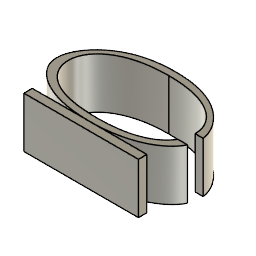
goulotte câbles (Autodesk Fusion 360 design; units mm, degrees)
Autodesk Fusion 360 part; units mm, degrees
sketch "Esquisse1" plane through (0, 0, 0) normal (0, 0, 1) x (1, 0, 0)
  line L0 (0, 0) -> (-17, 0)
  line L1 (-17, 0) -> (-17, 2.5)
  line L2 (-17, 2.5) -> (0, 2.5)
  spline S0 degree 5 poles (0, 2.5) (-1.0965, 2.5) (-3.2261, 2.5598) (-6.2303, 2.8288) (-9.8493, 3.531) (-13.6923, 4.8943) (-16.8066, 6.6306) (-19.1448, 8.6248) (-20.6721, 10.7786) (-21.3856, 13.0364) (-21.3178, 15.3875) (-20.5097, 17.8225) (-18.9943, 20.3035) (-16.7753, 22.7185) (-13.8294, 24.8979) (-10.1172, 26.6515) (-6.4978, 27.5688) (-3.4001, 27.9216) (-1.1622, 28) (0, 28) knots 0 0 0 0 0 0 0.066667 0.133333 0.2 0.266667 0.333333 0.4 0.466667 0.533333 0.6 0.666667 0.733333 0.8 0.866667 0.933333 1 1 1 1 1 1
  line L3 (0, 1.75) -> (0, 22.5)
  spline S1 degree 5 poles (0, 2.5) (1.0965, 2.5) (3.2261, 2.5598) (6.2303, 2.8288) (9.8493, 3.531) (13.6923, 4.8943) (16.8066, 6.6306) (19.1448, 8.6248) (20.6721, 10.7786) (21.3856, 13.0364) (21.3178, 15.3875) (20.5097, 17.8225) (18.9943, 20.3035) (16.7753, 22.7185) (13.8294, 24.8979) (10.1172, 26.6515) (6.4978, 27.5688) (3.4001, 27.9216) (1.1622, 28) (0, 28) knots 0 0 0 0 0 0 0.066667 0.133333 0.2 0.266667 0.333333 0.4 0.466667 0.533333 0.6 0.666667 0.733333 0.8 0.866667 0.933333 1 1 1 1 1 1
  line L4 (5.5634, 2.5) -> (-5.5634, 2.5)
  line L5 (-5.6976, 28) -> (5.6976, 28)
  line L6 (-5.5634, 2.5) -> (5.5634, 2.5)
  line L7 (5.6976, 28) -> (-5.6976, 28)
  line L8 (17, 2.5) -> (0, 2.5)
  line L9 (17, 0) -> (17, 2.5)
  line L10 (0, 0) -> (17, 0)
  spline S2 degree 5 poles (0, 4.5) (-0.9387, 4.5) (-2.7577, 4.5381) (-5.3111, 4.7097) (-8.3672, 5.1669) (-11.6138, 6.1149) (-14.2899, 7.4272) (-16.3901, 9.079) (-17.8969, 11.0271) (-18.7777, 13.2009) (-18.9888, 15.5036) (-18.4869, 17.8249) (-17.2389, 20.0482) (-15.2396, 22.061) (-12.5063, 23.7593) (-9.0653, 25.051) (-5.7682, 25.6992) (-2.9986, 25.9453) (-1.0213, 26) (0, 26) knots 0 0 0 0 0 0 0.066667 0.133333 0.2 0.266667 0.333333 0.4 0.466667 0.533333 0.6 0.666667 0.733333 0.8 0.866667 0.933333 1 1 1 1 1 1
  line L11 (5.5569, 4.5) -> (-5.5569, 4.5)
  line L12 (-5.6998, 26) -> (5.6998, 26)
  line L13 (1.75, 0) -> (22.5, 0)
  line L14 (0, 2.5) -> (0, 4.5)
  line L15 (0, 26) -> (0, 28)
  spline S3 degree 5 poles (0, 4.5) (0.9387, 4.5) (2.7577, 4.5381) (5.3111, 4.7097) (8.3672, 5.1669) (11.6138, 6.1149) (14.2899, 7.4272) (16.3901, 9.079) (17.8969, 11.0271) (18.7777, 13.2009) (18.9888, 15.5036) (18.4869, 17.8249) (17.2389, 20.0482) (15.2396, 22.061) (12.5063, 23.7593) (9.0653, 25.051) (5.7682, 25.6992) (2.9986, 25.9453) (1.0213, 26) (0, 26) knots 0 0 0 0 0 0 0.066667 0.133333 0.2 0.266667 0.333333 0.4 0.466667 0.533333 0.6 0.666667 0.733333 0.8 0.866667 0.933333 1 1 1 1 1 1
  line L16 (-5.5569, 4.5) -> (5.5569, 4.5)
  line L17 (5.6998, 26) -> (-5.6998, 26)
  point P0 (-20, 10)
  point P1 (-19.992, 18.499)
  point P2 (20, 10)
  point P3 (19.992, 18.499)
  point P4 (-17, 10)
  point P5 (-17.992, 18.499)
  point P6 (17, 10)
  point P7 (17.992, 18.499)
  dimension "d1" = 17
  dimension "d3" = 2.5
  dimension "d8" = 28
  dimension "d9" = 20
  dimension "d10" = 19.992
  dimension "d11" = 2
  dimension "d12" = 17
  dimension "d14" = 17.992
  dimension "d15" = 26
  constraint coincident L0.start L10.start
  constraint horizontal L0
  constraint perpendicular L0 L1
  constraint perpendicular L1 L2
  constraint coincident L2.end L3
  constraint midpoint L2.end L4
  constraint midpoint S0.end L5
  constraint symmetric L0.start L3 L10.start
  constraint symmetric L0.end L3 L9.start
  constraint symmetric L1.end L3 L8.start
  constraint symmetric L2.end L3 S0.start
  constraint symmetric P0 L3 P2
  constraint symmetric P1 L3 P3
  constraint symmetric S0.end L3 S1.end
  constraint symmetric L3 L4.start L4.end
  constraint symmetric L3 L4.end L4.start
  constraint symmetric L3 L5.start L5.end
  constraint symmetric L3 L5.end L5.start
  constraint midpoint S2.start L11
  constraint midpoint S2.end L12
  constraint horizontal P0 P4
  constraint horizontal P1 P5
  constraint perpendicular L8 L14
  constraint vertical L15
  constraint symmetric L3 P4 P6
  constraint symmetric L3 P5 P7
  constraint symmetric L3 S2.end L15.start
  constraint symmetric L3 S2.start L14.end
  constraint symmetric L3 L11.end L11.start
  constraint symmetric L3 L12.start L12.end
  constraint symmetric L3 L11.start L11.end
  constraint symmetric L3 L12.end L12.start
  constraint coincident L4.start L6.end
  constraint coincident L11.start L16.end
  constraint coincident L12.end L17.start
  constraint coincident L5.end L7.start
  measures "d1" distance of L0.start L0.end
  measures "d3" distance of L0.end L1.end
  measures "d8" distance of L0 S0.end
  measures "d9" distance of P0 L3
  measures "d10" distance of P1 L3
  measures "d11" distance of L2.end S2.start
  measures "d12" distance of L3 P4
  measures "d14" distance of L3 P5
  measures "d15" distance of S2.end L13
extrude "Extrusion2" add sketch "Esquisse1" along normal mid plane 15 contours S0 L3 S2 L14 L15 | L3 S1 L14 L15 S3 | L0 L1 L2 L4 L6 L8 L9 L10 L13
sketch "Esquisse2" plane through (0, 0, 7.5) normal (0, 0, 1) x (-1, 0, 0)
  spline S0 degree 5 poles (0, -26) (-1.0213, -26) (-2.9986, -25.9453) (-5.7682, -25.6992) (-9.0653, -25.051) (-12.5063, -23.7593) (-15.2396, -22.061) (-17.2389, -20.0482) (-18.4869, -17.8249) (-18.9888, -15.5036) (-18.7777, -13.2009) (-17.8969, -11.0271) (-16.3901, -9.079) (-14.2899, -7.4272) (-11.6138, -6.1149) (-8.3672, -5.1669) (-5.3111, -4.7097) (-2.7577, -4.5381) (-0.9387, -4.5) (0, -4.5) knots -1 -1 -1 -1 -1 -1 -0.933333 -0.866667 -0.8 -0.733333 -0.666667 -0.6 -0.533333 -0.466667 -0.4 -0.333333 -0.266667 -0.2 -0.133333 -0.066667 0 0 0 0 0 0
  spline S1 degree 5 poles (0, -4.5) (0.9387, -4.5) (2.7577, -4.5381) (5.3111, -4.7097) (8.3672, -5.1669) (11.6138, -6.1149) (14.2899, -7.4272) (16.3901, -9.079) (17.8969, -11.0271) (18.7777, -13.2009) (18.9888, -15.5036) (18.4869, -17.8249) (17.2389, -20.0482) (15.2396, -22.061) (12.5063, -23.7593) (9.0653, -25.051) (5.7682, -25.6992) (2.9986, -25.9453) (1.0213, -26) (0, -26) knots 0 0 0 0 0 0 0.066667 0.133333 0.2 0.266667 0.333333 0.4 0.466667 0.533333 0.6 0.666667 0.733333 0.8 0.866667 0.933333 1 1 1 1 1 1
  spline S2 degree 5 poles (0, -2.5) (-1.0965, -2.5) (-3.2261, -2.5598) (-6.2303, -2.8288) (-9.8493, -3.531) (-13.6923, -4.8943) (-16.8066, -6.6306) (-19.1448, -8.6248) (-20.6721, -10.7786) (-21.3856, -13.0364) (-21.3178, -15.3875) (-20.5097, -17.8225) (-18.9943, -20.3035) (-16.7753, -22.7185) (-13.8294, -24.8979) (-10.1172, -26.6515) (-6.4978, -27.5688) (-3.4001, -27.9216) (-1.1622, -28) (0, -28) knots 0 0 0 0 0 0 0.066667 0.133333 0.2 0.266667 0.333333 0.4 0.466667 0.533333 0.6 0.666667 0.733333 0.8 0.866667 0.933333 1 1 1 1 1 1
  spline S3 degree 5 poles (0, -28) (1.1622, -28) (3.4001, -27.9216) (6.4978, -27.5688) (10.1172, -26.6515) (13.8294, -24.8979) (16.7753, -22.7185) (18.9943, -20.3035) (20.5097, -17.8225) (21.3178, -15.3875) (21.3856, -13.0364) (20.6721, -10.7786) (19.1448, -8.6248) (16.8066, -6.6306) (13.6923, -4.8943) (9.8493, -3.531) (6.2303, -2.8288) (3.2261, -2.5598) (1.0965, -2.5) (0, -2.5) knots -1 -1 -1 -1 -1 -1 -0.933333 -0.866667 -0.8 -0.733333 -0.666667 -0.6 -0.533333 -0.466667 -0.4 -0.333333 -0.266667 -0.2 -0.133333 -0.066667 0 0 0 0 0 0
  line L0 (-23, -15) -> (-11, -15)
  line L1 (-11, -15) -> (-11, -11)
  line L2 (-11, -11) -> (-23, -11)
  line L3 (-23, -11) -> (-23, -15)
  line L4 (-23, -15) -> (-11, -11) construction
  line L5 (-11, -15) -> (-23, -11) construction
  point P0 (-17, -13)
  dimension "d20" = 4
  constraint horizontal L0
  constraint perpendicular L0 L1
  constraint parallel L0 L2
  constraint parallel L1 L3
  constraint coincident L4 P0
  constraint coincident L5 P0
  measures "d20" distance of L0.start L2.end
extrude "Extrusion3" cut sketch "Esquisse2" against normal blind 15 contours S0 S2 L0 L2
